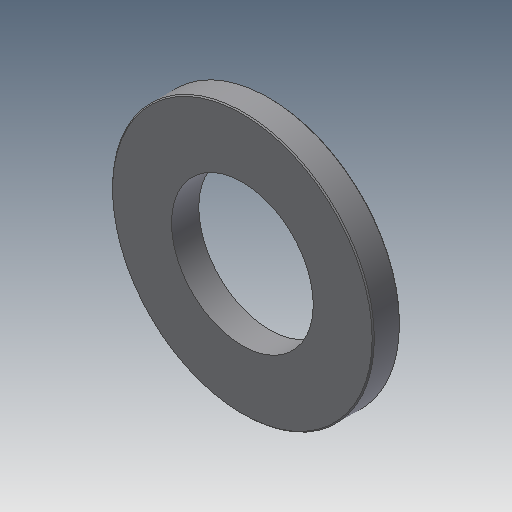
# Autodesk Inventor part: M12 rodela
Saved by Autodesk Inventor 2018 (Build 220112000, 112)
## iProperties
Created: 2014-11-19
Part Number: M12 rodela
Document SubType Name: Modeling
Designer: support
Manufacturer: Standard
Standards Organization: Custom
Material: Generic
Density: 1 g/cm^3
Appearance: Default
Author: support
Autodesk Inventor part; units mm, degrees
ref_plane "YZ Plane" through (0, 0, 0) normal (1, 0, 0) x (0, 1, 0)
ref_plane "XZ Plane" through (0, 0, 0) normal (0, 1, 0) x (-1, 0, 0)
ref_plane "XY Plane" through (0, 0, 0) normal (0, 0, 1) x (1, 0, 0)
sketch "Sketch1" plane through (0, 0, 0) normal (0, 0, 1) x (1, 0, 0)
  circle A0 centre (0, 0) radius 12
  circle A1 centre (0, 0) radius 6.5
  dimension "d0" = 13
  dimension "d1" = 24
  constraints: 2 centre point, 1 coincident
  measures "d0" diameter of A1
  measures "d1" diameter of A0
extrude "Extrusion1" add sketch "Sketch1" along normal blind 2.5
chamfer "Chamfer1" distance 0.1 angle 45 2 edges at (-12, 0, 2.5) (-12, 0, 0)
body "Solid1"
